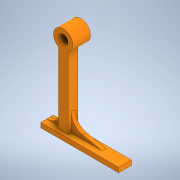
# Autodesk Inventor part: Stand
Saved by Autodesk Inventor 2020.3 (Build 243373000, 373)
## iProperties
Created: 2021-06-11
Part Number: Stand
Material: Steel, Mild
Document SubType Name: Modeling
Designer: User
Density: 7.85 g/cm^3
Appearance: Orange
Mass: 167.623 g
Surface Area: 98.1801 cm^2
Volume: 21.3533 cm^3
Author: User
Autodesk Inventor part; units mm, degrees
ref_plane "YZ Plane" through (0, 0, 0) normal (1, 0, 0) x (0, 1, 0)
ref_plane "XZ Plane" through (0, 0, 0) normal (0, 1, 0) x (-1, 0, 0)
sketch "Sketch1" plane through (0, 0, 0) normal (0, 0, 1) x (1, 0, 0)
  line L0 (0, 0) -> (0, -15) construction
  line L1 (-5, 0) -> (-5, -15)
  line L2 (5, -15) -> (5, 0)
  arc A0 (5, 0) -> (-5, 0) centre (0, 0) ccw
  arc A1 (-5, -15) -> (5, -15) centre (0, -15) ccw
  line L3 (0, 0) -> (0, -15) construction
  line L4 (-10, 0) -> (-10, -15)
  line L5 (10, -15) -> (10, 0)
  arc A2 (10, 0) -> (-10, 0) centre (0, 0) ccw
  line L6 (0, -15) -> (0, -87) construction
  line L7 (5, -23.6603) -> (5, -82)
  line L8 (-5, -23.6603) -> (-5, -82)
  arc A3 (-10, -15) -> (-5, -23.6603) centre (0, -15) ccw
  arc A4 (5, -23.6603) -> (10, -15) centre (0, -15) ccw
  line L9 (-20, -82) -> (60, -82)
  line L10 (60, -82) -> (60, -87)
  line L11 (60, -87) -> (-20, -87)
  line L12 (-20, -87) -> (-20, -82)
  circle A5 centre (0, 0) radius 5
  circle A6 centre (0, 0) radius 10
  line L13 (-5, -23.6603) -> (-5, 8.6603)
  line L14 (5, -23.6603) -> (5, 8.6603)
  point P0 (0, -7.5)
  point P1 (0, -7.5)
  point P2 (5, 0)
  point P3 (5, -8.6603)
  point P4 (-5, -8.6603)
  dimension "d0" = 15
  dimension "d1" = 5
  dimension "d2" = 10
  dimension "d3" = 72
  dimension "d4" = 5
  dimension "d5" = 5
  dimension "d7" = 80
  dimension "d8" = 5
  dimension "d24" = 15
  constraints: 34 end point, 12 point on circle, 10 tangent, 7 centre point, 6 parallel, 4 vertical, 2 coincident, 2 midpoint, 2 point on line, 1 collinear, 1 horizontal, 1 perpendicular
  measures "d0" distance of L0.end L0.start
  measures "d1" distance of L1.end L0.end
  measures "d2" distance of L4.end L0.end
  measures "d3" distance of L0.end L6.end
  measures "d4" distance between parallel lines of L6 L7
  measures "d5" distance between parallel lines of L6 L8
  measures "d7" distance of L10.end L11.end
  measures "d8" distance of L9.end L10.end
  measures "d24" distance of L9.start L8.end
extrude "Extrusion1" add sketch "Sketch1" along normal blind 10 contours A5 L2 A6 L1 | L13 A2 L14 A0 | L1 A6 A2 L13 | A6 L2 A1 L1 | L14 A2 A6 L2 | A1 L14 L7 L9 L8 L13 | L9 L10 L11 L12
sketch "Sketch2" plane through (0, 0, 0) normal (0, 0, -1) x (-1, 0, 0)
  arc A0 (-5, -15) -> (5, -15) centre (0, -15) ccw projected
  line L0 (0, 0) -> (0, -15) construction
  line L1 (-10, 0) -> (-10, -15)
  line L2 (10, -15) -> (10, 0)
  arc A1 (10, 0) -> (-10, 0) centre (0, 0) ccw
  arc A2 (-10, -15) -> (10, -15) centre (0, -15) ccw
  line L3 (0, 0) -> (0, -15) construction
  line L4 (-5, 0) -> (-5, -15)
  line L5 (5, -15) -> (5, 0)
  arc A3 (5, 0) -> (-5, 0) centre (0, 0) ccw
  arc A4 (-5, -15) -> (5, -15) centre (0, -15) ccw
  circle A5 centre (0, 0) radius 10
  circle A6 centre (0, 0) radius 5
  point P0 (0, -7.5)
  point P1 (0, -7.5)
  point P2 (-5, -15)
  dimension "d11" = 10
  dimension "d12" = 5
  constraints: 16 end point, 8 point on circle, 8 tangent, 5 centre point, 3 equal length, 2 coincident, 2 midpoint, 1 vertical, 3 other
  measures "d11" distance of L2.end L0.start
  measures "d12" distance of L0.start L5.end
extrude "Extrusion2" add sketch "Sketch2" along normal blind 8 contours A5 A1 L5 A3 L4 | L4 A6 L5 A5
sketch "Sketch3" plane through (0, 0, 10) normal (0, 0, 1) x (1, 0, 0)
  line L0 (-20, -82) -> (-20, -87) projected
  line L1 (-20, -87) -> (60, -87) projected
  line L2 (-20, -82) -> (60, -82)
  line L3 (60, -82) -> (60, -87)
  line L4 (60, -87) -> (-20, -87)
  line L5 (-20, -87) -> (-20, -82)
  point P0 (0, 0)
  dimension "d23" = 80
  constraints: 8 end point, 2 parallel, 1 horizontal, 1 perpendicular
  measures "d23" distance of L0.end L1.end
extrude "Extrusion3" add sketch "Sketch3" along normal blind 3
ref_plane "Work Plane1" through (0, 0, 5) normal (0, 0, 1) x (1, 0, 0)
sketch "Sketch4" plane through (0, 0, 5) normal (0, 0, 1) x (1, 0, 0)
  arc A0 (-20, -82) -> (-5, -67) centre (-20, -67) ccw
  line L0 (-5, -23.6603) -> (-5, -82) projected
  line L1 (60, -82) -> (-20, -82) projected
  line L2 (-5, -67) -> (-20, -67) construction
  line L3 (-20, -67) -> (-20, -82) construction
  line L4 (-20, -82) -> (-5, -82)
  line L5 (-5, -82) -> (-5, -67)
  arc A1 (5, -63) -> (16.8392, -77.6632) centre (20, -63) ccw
  line L6 (5, -82) -> (5, -23.6603) projected
  line L7 (16.8392, -77.6632) -> (36.9579, -82)
  line L8 (5, -82) -> (5, -63)
  point P0 (0, 0)
  point P1 (-20, -82)
  dimension "d17" = 15
  dimension "d18" = 30
  dimension "d20" = 19
  constraints: 12 end point, 4 point on circle, 4 tangent, 3 point on line, 2 centre point, 2 parallel, 2 perpendicular
  measures "d17" radius of A0
  measures "d18" diameter of A1
  measures "d20" distance from line of L1 A1.centre
extrude "Extrusion4" add sketch "Sketch4" along normal mid plane 4
equation "\"d9\" = d2"
body "Solid1"
